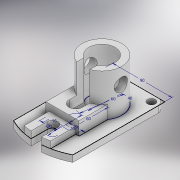
# Autodesk Inventor part: 2020216649-唐晨超-组合体1-2
Saved by Autodesk Inventor 2020 (Build 240168000, 168)
## iProperties
Created: 2021-03-17
Part Number: 2020216649-唐晨超-组合体1-2
Material: 常规
Document SubType Name: Modeling
Designer: Luorily
Density: 1 g/cm^3
Appearance: 默认
Author: Luorily
Autodesk Inventor part; units mm, degrees
ref_plane "YZ Plane" through (0, 0, 0) normal (1, 0, 0) x (0, 1, 0)
ref_plane "XZ Plane" through (0, 0, 0) normal (0, 1, 0) x (-1, 0, 0)
ref_plane "XY Plane" through (0, 0, 0) normal (0, 0, 1) x (1, 0, 0)
sketch "草图1" plane through (0, 0, 0) normal (0, 1, 0) x (-1, 0, 0)
  line L0 (45, -50) -> (-45, -50)
  line L1 (-45, -50) -> (-45, 89.3029)
  line L2 (45, -50) -> (45, 89.3029)
  circle A0 centre (0, 0) radius 20
  arc A1 (-10, 28.2843) -> (10, 28.2843) centre (0, 0) ccw
  arc A2 (-8, 75) -> (8, 75) centre (0, 75) ccw
  line L3 (8, 75) -> (8, 99.6795)
  line L4 (-8, 75) -> (-8, 99.6795)
  arc A3 (-8, 99.6795) -> (-45, 89.3029) centre (0, 0) ccw
  arc A4 (45, 89.3029) -> (8, 99.6795) centre (0, 0) ccw
  line L5 (0, 60) -> (25, 60)
  line L6 (25, 60) -> (25, 16.5831)
  line L7 (0, 60) -> (-25, 60)
  line L8 (-25, 60) -> (-25, 16.5831)
  arc A5 (10, 40) -> (-10, 40) centre (0, 40) ccw
  line L9 (-10, 40) -> (-10, 28.2843)
  line L10 (10, 40) -> (10, 28.2843)
  line L11 (0, 60) -> (20, 60)
  line L12 (20, 60) -> (20, 97.9796)
  line L13 (0, 60) -> (-20, 60)
  line L14 (-20, 60) -> (-20, 97.9796)
  line L15 (10, 28.2843) -> (10, 17.3205)
  line L16 (-10, 28.2843) -> (-10, 17.3205)
  dimension "d3" = 90
  dimension "d4" = 40
  dimension "d5" = 60
  dimension "d7" = 16
  dimension "d20" = 60
  dimension "d21" = 25
  dimension "d22" = 25
  dimension "d24" = 20
  dimension "d29" = 20
  dimension "d30" = 20
  constraints: 34 end point, 16 point on circle, 6 centre point, 5 perpendicular, 4 vertical, 3 coincident, 2 parallel, 2 point on line, 1 horizontal, 1 tangent
  measures "d3" distance of L0.start L0.end
  measures "d4" diameter of A0
  measures "d5" diameter of A1
  measures "d7" diameter of A2
  measures "d20" distance of A1.centre L5.start
  measures "d21" distance of L5.start L5.end
  measures "d22" distance of L5.start L7.end
  measures "d24" diameter of A5
  measures "d29" distance of L5.start L11.end
  measures "d30" distance of L5.start L13.end
extrude "拉伸1" add sketch "草图1" against normal blind 10
extrude "拉伸2" add sketch "草图1" along normal blind 64 contours A1 L16 A0 L15
sketch "草图2" plane through (45, 0, 89.3029) normal (1, 0, 0) x (0, 0, -1)
  line L0 (89.3029, 0) -> (89.3029, 40)
  dimension "d12" = 40
  constraints: 2 end point, 1 vertical
  measures "d12" distance of L0.start L0.end
hole "孔1" at (45, 40, 0) direction (-1, 0, 0) diameter 20 end through all
extrude "拉伸3" add sketch "草图1" along normal blind 20 contours L5 L6 A1 L10 A5 L9 L8 L7
extrude "拉伸4" add sketch "草图1" along normal blind 5 contours L15 A0 L16 L9 A5 L10
extrude "拉伸5" add sketch "草图1" along normal blind 10 contours L12 L5 L7 L14 A3 L4 A2 L3 A4
fillet "圆角1" radius 10 2 edges at (45, -5, -50) (-45, -5, -50)
sketch "草图3" plane through (0, 0, 0) normal (0, 1, 0) x (1, 0, 0)
  arc A0 (-35, 50) -> (-45, 40) centre (-35, 40) ccw projected
  arc A1 (45, 40) -> (35, 50) centre (35, 40) ccw projected
  constraints: 2 coincident
hole "孔2" at (-35, 0, -40) at (35, 0, -40) direction (0, -1, 0) diameter 12 end through all
